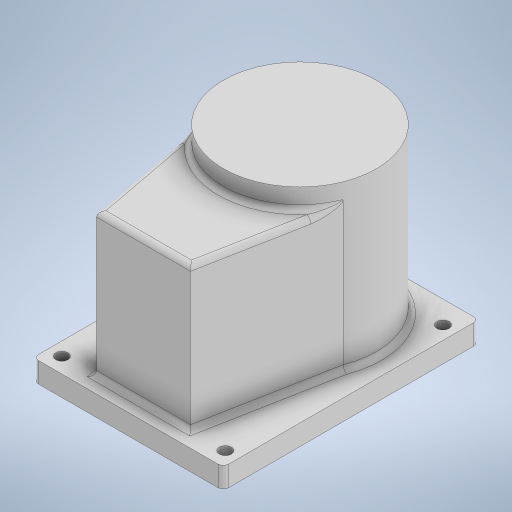
# Autodesk Inventor part: part7
Saved by Autodesk Inventor 2024 (Build 280153000, 153)
## iProperties
Created: 2023-08-22
Part Number: part7
Material: Generic
Document SubType Name: Modeling
Designer: admins
Density: 1 g/cm^3
Appearance: Default
Author: admins
Autodesk Inventor part; units mm, degrees
ref_plane "YZ Plane" through (0, 0, 0) normal (1, 0, 0) x (0, 1, 0)
ref_plane "XZ Plane" through (0, 0, 0) normal (0, 1, 0) x (-1, 0, 0)
ref_plane "XY Plane" through (0, 0, 0) normal (0, 0, 1) x (1, 0, 0)
sketch "Sketch1" plane through (0, 0, 0) normal (0, 1, 0) x (-1, 0, 0)
  line L0 (10.3645, 25.8906) -> (-175.6355, 25.8906)
  line L1 (-175.6355, 25.8906) -> (-175.6355, -224.1094)
  line L2 (-175.6355, -224.1094) -> (10.3645, -224.1094)
  line L3 (10.3645, -224.1094) -> (10.3645, 25.8906)
  point P0 (0, 0)
  dimension "d0" = 186
  dimension "d1" = 250
  constraints: 8 end point, 2 parallel, 1 horizontal, 1 perpendicular
  measures "d0" distance of L2.end L1.end
  measures "d1" distance of L1.end L0.end
extrude "Extrusion1" add sketch "Sketch1" along normal blind 180
sketch "Sketch2" plane through (0, 180, 0) normal (0, 1, 0) x (1, 0, 0)
  circle A0 centre (82.6355, 142.1094) radius 75
  line L0 (175.6355, 224.1094) -> (-10.3645, 224.1094) projected
  line L1 (36.6355, -10.8906) -> (128.6355, -10.8906)
  line L2 (128.6355, -10.8906) -> (152.4335, 114.664)
  line L3 (36.6355, -10.8906) -> (12.8376, 114.664)
  circle A1 centre (162.6355, -10.8906) radius 6
  circle A2 centre (2.6355, -10.8906) radius 6
  line L4 (175.6355, -25.8906) -> (175.6355, 224.1094) projected
  circle A3 centre (162.6355, 202.1094) radius 6
  circle A4 centre (2.6355, 202.1094) radius 6
  line L5 (-10.3645, -25.8906) -> (175.6355, -25.8906)
  line L6 (175.6355, -25.8906) -> (175.6355, 224.1094)
  line L7 (175.6355, 224.1094) -> (-10.3645, 224.1094)
  line L8 (-10.3645, 224.1094) -> (-10.3645, -25.8906)
  point P0 (0, 0)
  dimension "d4" = 150
  dimension "d9" = 92
  dimension "d11" = 12
  dimension "d16" = 12
  constraints: 14 end point, 5 centre point, 2 horizontal, 2 parallel, 2 point on circle, 1 perpendicular
  measures "d4" diameter of A0
  measures "d9" distance of L1.start L1.end
  measures "d11" diameter of A1
  measures "d16" diameter of A4
extrude "Extrusion2" cut sketch "Sketch2" against normal blind 20 contours A0 L2 L1 L3
extrude "Extrusion3" cut sketch "Sketch2" against normal blind 160
extrude "Extrusion4" cut sketch "Sketch2" against normal blind 200 contours A2
extrude "Extrusion5" cut sketch "Sketch2" against normal blind 200 contours A1
extrude "Extrusion6" cut sketch "Sketch2" against normal blind 200 contours A4
extrude "Extrusion7" cut sketch "Sketch2" against normal blind 200 contours A3
fillet "Fillet1" radius 5 12 edges at (140.5345, 160, -51.8867) (140.5345, 20, -51.8867) (82.6355, 160, 10.8906) (24.7365, 160, -51.8867) (24.7365, 20, -51.8867) (82.6355, 20, 10.8906) (82.6355, 160, -67.1094) (175.6355, 10, 25.8906) (175.6355, 10, -224.1094) (-10.3645, 10, 25.8906) (-10.3645, 10, -224.1094) (82.6355, 20, -217.1094)
body "Solid1"
